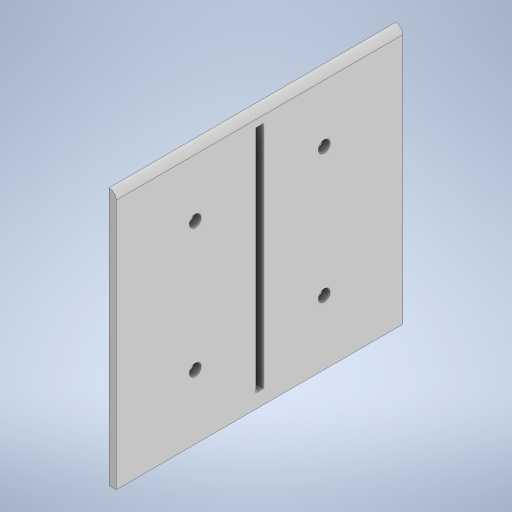
# Autodesk Inventor part: Gripper plate
Saved by Autodesk Inventor 2023 (Build 270158000, 158)
## iProperties
Created: 2023-02-27
Part Number: Gripper plate
Material: Generic
Document SubType Name: Modeling
Designer: Gabriel - T3 CAD
Density: 1 g/cm^3
Appearance: Default
Author: Gabriel - T3 CAD
Autodesk Inventor part; units mm, degrees
ref_plane "YZ Plane" through (0, 0, 0) normal (1, 0, 0) x (0, 1, 0)
ref_plane "XZ Plane" through (0, 0, 0) normal (0, 1, 0) x (-1, 0, 0)
ref_plane "XY Plane" through (0, 0, 0) normal (0, 0, 1) x (1, 0, 0)
sketch "Sketch1" plane through (0, 0, 0) normal (1, 0, 0) x (0, 1, 0)
  line L0 (0, 0) -> (-127, 0)
  line L1 (-127, 0) -> (-127, 127)
  line L2 (-127, 127) -> (0, 127)
  line L3 (0, 127) -> (0, 0)
  line L4 (-19.05, 65.151) -> (-120.65, 65.151)
  line L5 (-120.65, 65.151) -> (-120.65, 61.849)
  line L6 (-120.65, 61.849) -> (-19.05, 61.849)
  line L7 (-19.05, 61.849) -> (-19.05, 65.151)
  line L8 (0, 47.625) -> (-12.7, 47.625)
  line L9 (-12.7, 47.625) -> (-12.7, 79.375)
  line L10 (-12.7, 79.375) -> (0, 79.375)
  line L11 (0, 79.375) -> (0, 47.625)
  line L12 (-12.7, 47.625) -> (-12.7, 0)
  line L13 (-12.7, 79.375) -> (-12.7, 127)
  dimension "d0" = 127
  dimension "d1" = 127
  dimension "d2" = 6.35
  dimension "d4" = 3.302
  dimension "d5" = 61.849
  dimension "d25" = 12.7
  dimension "d26" = 31.75
  dimension "d27" = 47.625
  dimension "d28" = 6.35
  constraints: 28 end point, 6 parallel, 4 perpendicular, 4 point on line, 3 horizontal
  measures "d0" distance of L1.end L2.end
  measures "d1" distance of L0.end L1.end
  measures "d2" distance between parallel lines of L1 L5
  measures "d4" distance between parallel lines of L6 L4
  measures "d5" distance between parallel lines of L0 L6
  measures "d25" distance of L8.start L8.end
  measures "d26" distance of L8.end L9.end
  measures "d27" distance between parallel lines of L0 L8
  measures "d28" distance between parallel lines of L9 L7
extrude "Extrusion1" add sketch "Sketch1" along normal blind 3.175 contours L0 L1 L2 L13 L9 L12
sketch "Sketch3" plane through (0, 0, 0) normal (-1, 0, 0) x (0, 0, 1)
  circle A0 centre (34.925, -41.275) radius 2.5797
  line L0 (0, -127) -> (0, -12.7) projected
  line L1 (0, -12.7) -> (0, 0)
  line L2 (0, 0) -> (20.4302, 0)
  line L3 (20.4302, 0) -> (0, -12.7)
  circle A1 centre (34.925, -98.425) radius 2.5797
  circle A2 centre (92.075, -41.275) radius 2.5797
  circle A3 centre (92.075, -98.425) radius 2.5797
  line L4 (0, -12.7) -> (127, -12.7) projected
  dimension "d31" = 57.15
  dimension "d34" = 57.15
  dimension "d37" = 34.925
  dimension "d38" = 28.575
  dimension "d39" = 5.1594
  constraints: 6 end point, 4 centre point, 1 collinear, 1 horizontal, 1 perpendicular, 1 vertical, 6 other
  measures "d31" distance of A0.centre A1.centre
  measures "d34" distance of A0.centre A2.centre
  measures "d37" distance from line of L0 A0.centre
  measures "d38" distance from line of L4 A0.centre
  measures "d39" diameter of A0
extrude "Extrusion4" cut sketch "Sketch3" against normal through all contours A0 | A1 | A2 | A3
fillet "Fillet5" radius 3.175 1 edges at (3.175, -12.7, 63.5)
equation "\"d5\" = -0.5 * d4 + 0.5 * d1"
equation "\"d27\" = -0.5 * d26 + 0.5 * d1"
equation "\"d28\" = d2"
body "Solid1"
